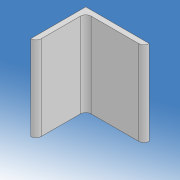
# Autodesk Inventor part: NASA-20-EBOX-EXT-CB-01
Saved by Autodesk Inventor 2020 (Build 240168000, 168)
## iProperties
Created: 2019-12-04
Part Number: NASA-20-EBOX-EXT-CB-01
Material: Generic
Document SubType Name: Modeling
Designer: mpark
Density: 1 g/cm^3
Appearance: Default
Author: mpark
Autodesk Inventor part; units mm, degrees
ref_plane "YZ Plane" through (0, 0, 0) normal (1, 0, 0) x (0, 1, 0)
ref_plane "XZ Plane" through (0, 0, 0) normal (0, 1, 0) x (-1, 0, 0)
ref_plane "XY Plane" through (0, 0, 0) normal (0, 0, 1) x (1, 0, 0)
sketch "Sketch1" plane through (0, 0, 0) normal (0, 1, 0) x (-1, 0, 0)
  line L0 (-38.1, 0) -> (0, 0)
  line L1 (0, 0) -> (0, 33.02)
  line L2 (-34.925, 3.175) -> (-6.35, 3.175)
  line L3 (-3.175, 6.35) -> (-3.175, 29.845)
  line L4 (0, 33.02) -> (0, 33.02)
  line L5 (-38.1, 0) -> (-38.1, 0)
  arc A0 (0, 33.02) -> (-3.175, 29.845) centre (0, 29.845) ccw
  arc A1 (-34.925, 3.175) -> (-38.1, 0) centre (-34.925, 0) ccw
  arc A2 (-6.35, 3.175) -> (-3.175, 6.35) centre (-6.35, 6.35) ccw
  dimension "d0" = 33.02
  dimension "d1" = 38.1
  dimension "d2" = 3.175
  dimension "d3" = 3.175
  constraints: 12 end point, 6 point on circle, 6 tangent, 3 centre point, 3 perpendicular, 2 equal radius, 2 horizontal, 1 other
  measures "d0" distance of L0.end L1.end
  measures "d1" distance of L0.start L0.end
  measures "d2" distance between parallel lines of L0 L2
  measures "d3" radius of A0
extrude "Extrusion1" add sketch "Sketch1" along normal blind 50.8
body "Solid1"
